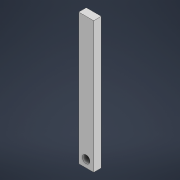
# Autodesk Inventor part: Cube_Holder_SB_V1_(71mm)
Saved by Autodesk Inventor 2022 (Build 260153000, 153)
## iProperties
Created: 2023-05-10
Part Number: Cube_Holder_SB_V1_(71mm)
Material: Generic
Document SubType Name: Modeling
Designer: Karl Spiteri
Density: 1 g/cm^3
Appearance: Default
Author: Karl Spiteri
Autodesk Inventor part; units mm, degrees
ref_plane "YZ Plane" through (0, 0, 0) normal (1, 0, 0) x (0, 1, 0)
ref_plane "XZ Plane" through (0, 0, 0) normal (0, 1, 0) x (-1, 0, 0)
ref_plane "XY Plane" through (0, 0, 0) normal (0, 0, 1) x (1, 0, 0)
sketch "Sketch2" plane through (0, 0, 0) normal (0, 0, 1) x (1, 0, 0)
  line L0 (0, 0) -> (-9.9, 0)
  line L1 (-4.95, 0) -> (-4.95, 2.5)
  line L2 (-4.95, 0) -> (-2.45, 0) construction
  circle A0 centre (-4.95, 5) radius 2.5
  line L3 (-4.95, 7.5) -> (32.05, 7.5) construction
  line L4 (0, 0) -> (-9.9, 0)
  line L5 (0, 0) -> (-9.9, 0)
  line L6 (-4.95, 7.5) -> (66.05, 7.5) construction
  line L7 (-4.95, 7.5) -> (70.05, 7.5) construction
  line L8 (0, 0) -> (-9.9, 0)
  line L9 (-9.9, 0) -> (-9.9, 82.5)
  line L10 (0, 82.5) -> (0, 0)
  line L11 (-4.95, 7.5) -> (74.05, 7.5) construction
  line L12 (-9.9, 86.5) -> (0, 86.5)
  line L13 (0, 86.5) -> (0, 82.5)
  line L14 (-9.9, 82.5) -> (-9.9, 86.5)
  dimension "d35" = 5
  dimension "d33" = 2.5
  dimension "d34" = 90
  dimension "d48" = 9.9
  constraints: 30 end point, 8 horizontal, 3 perpendicular, 2 parallel, 1 midpoint, 1 point on line, 1 vertical, 1 vertical alignment, 2 other
  measures "d33" distance of L1.start L1.end
  measures "d34" angle of L2 L1
  measures "d48" distance of L9.end L10.start
extrude "Extrusion7" add sketch "Sketch2" along normal blind 5
body "Solid6"
